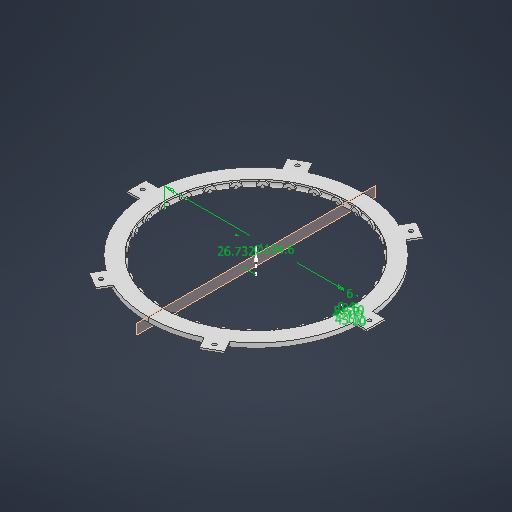
# Autodesk Inventor part: SAFRS-P-0034
Saved by Autodesk Inventor 2026.2 (Build 302298000, 298)
## iProperties
Created: 2025-12-01
Part Number: SAFRS-P-0034
Material: 일반
Document SubType Name: Modeling
Designer: jaewook
Density: 1 g/cm^3
Appearance: 기본값
Author: jaewook
Title: Fixer V1
Autodesk Inventor part; units mm, degrees
ref_plane "XZ Plane" through (0, 0, 0) normal (0, 1, 0) x (-1, 0, 0)
ref_plane "XY Plane" through (0, 0, 0) normal (0, 0, 1) x (1, 0, 0)
sketch "스케치1" plane through (0, 0, 0) normal (0, 0, 1) x (1, 0, 0)
  line L0 (0, 13.366) -> (0, -13.366)
  line L1 (98.7799, 5) -> (104.7799, 5)
  line L2 (104.7799, 5) -> (104.7799, -5)
  line L3 (104.7799, -5) -> (98.7799, -5)
  line L4 (98.7799, -5) -> (98.7799, 5)
  circle A0 centre (99.2799, 0) radius 3.1
  line L5 (99.2799, 0) -> (96.1799, 0)
  line L6 (96.1799, 7.3721) -> (96.1799, -2.237) construction
  line L7 (96.5799, 5) -> (96.5799, 1.5232)
  line L8 (96.5799, 5) -> (98.7799, 5)
  line L9 (99.7799, -5) -> (99.7799, -3.0594)
  circle A1 centre (99.2799, 0) radius 2.8 construction
  line L10 (99.3622, -4.0421) -> (90.1233, 5.1968) construction
  line L11 (99.2799, 0) -> (97.3, -1.9799) construction
  line L12 (104.7799, 0) -> (114.7799, 0)
  line L13 (114.7799, 0) -> (114.7799, 5)
  line L14 (114.7799, 5) -> (104.7799, 5)
  line L15 (104.7799, 5) -> (104.7799, 0)
  line L16 (99.7799, -3.0594) -> (101.7205, -5)
  point P0 (0, 0)
  point P1 (0, 0)
  point P2 (98.7799, 3.0594)
  dimension "d19" = 5.6
  dimension "d0" = 26.732
  dimension "d1" = 6.2
  dimension "d2" = 0.5
  dimension "d3" = 1
  dimension "d4" = 10
  dimension "d5" = 6
  dimension "d6" = 0.4
  dimension "d20" = 194.6
  dimension "d21" = 45
  dimension "d22" = 10
  dimension "d29" = 45
  constraints: 34 end point, 4 parallel, 4 vertical, 3 horizontal, 3 perpendicular, 3 point on circle, 3 point on line, 2 coincident, 2 horizontal alignment, 2 midpoint, 1 centre point, 1 collinear, 1 tangent, 4 other
  measures "d0" distance of L0.end L0.start
  measures "d1" diameter of A0
  measures "d2" distance from line of L5.start L4
  measures "d3" distance between parallel lines of L9 L4
  measures "d4" distance of L1.end L2.end
  measures "d5" distance of L1.start L1.end
  measures "d6" distance between parallel lines of L7 L6
  measures "d20" diameter of L11.end L0
  measures "d21" angle of L11 L5
  measures "d22" distance of L13.end L14.end
  measures "d29" angle of L3 L16
revolve "회전1" add sketch "스케치1" angle 360 about axis through (0, 13.366, 0) along (0, -1, 0) contours L1 L2 L3 L16 A0 L4 | L14 L13 L12 L2
revolve "회전2" add sketch "스케치1" angle 180 mid plane about axis through (99.2799, 0, 0) along (-1, 0, 0) contours L4 A0 L7 L8
pattern_circular "원형 패턴1" count 30 over 360 about axis through (0, -10, 0) along (0, 1, 0) of "회전2"
sketch "스케치7" plane through (0, 5, 0) normal (0, 1, 0) x (1, 0, 0)
  arc A0 (96.6213, -20.5375) -> (98.7799, 0) centre (0, 0) ccw projected
  circle A1 centre (0, 0) radius 114.7799 projected
  line L0 (114.7799, -10) -> (127.7799, -10)
  line L1 (127.7799, -10) -> (127.7799, 10)
  line L2 (127.7799, 10) -> (114.7799, 10)
  line L3 (114.7799, 10) -> (114.7799, -10) construction
  line L4 (114.7799, -10) -> (127.7799, 10) construction
  line L5 (127.7799, -10) -> (114.7799, 10) construction
  line L6 (114.7799, 10) -> (114.3435, 10)
  line L7 (114.7799, -10) -> (114.3435, -10)
  point P0 (121.2799, 0)
  dimension "d41" = 13
  dimension "d42" = 20
  constraints: 16 end point, 3 horizontal, 2 midpoint, 2 parallel, 2 point on circle, 1 horizontal alignment, 1 perpendicular, 1 tangent
  measures "d41" distance of L2.end L1.end
  measures "d42" distance of L1.end L0.end
extrude "돌출2" add sketch "스케치7" against normal blind 2 contours A1 L6 L2 L1 L0 L7
sketch "스케치3" plane through (0, 0, 0) normal (0, -1, 0) x (1, 0, 0)
  circle A0 centre (121.0617, 0) radius 2
  line L0 (127.7799, -10) -> (114.3435, -10) projected
  line L1 (127.7799, 10) -> (127.7799, -10) projected
  line L2 (114.3435, 10) -> (127.7799, 10) projected
  line L3 (114.3435, 10) -> (127.7799, -10) construction
  line L4 (114.3435, -10) -> (127.7799, 10) construction
  dimension "d23" = 4
  constraints: 4 end point, 2 coincident, 1 centre point, 1 midpoint
  measures "d23" diameter of A0
extrude "돌출1" cut sketch "스케치3" against normal through all
pattern_circular "원형 패턴3" count 6 over 360 about axis through (0, -10, 0) along (0, 1, 0) of "돌출1", "돌출2"
sketch "스케치2" plane through (0, 0, 0) normal (0, 0, 1) x (1, 0, 0)
  circle A0 centre (99.2799, 0) radius 3.1 projected
  circle A1 centre (99.2799, 0) radius 2.8
  line L0 (99.2799, -2.8) -> (99.2799, 2.8)
  line L1 (100.192, -3.6136) -> (93.7956, -0.336)
  line L2 (100.192, -3.6136) -> (94.0407, -3.6136)
  point P0 (0, 0)
  point P1 (98.003, -2.4919)
  dimension "d13" = 5.6
  dimension "d18" = 98.003
  constraints: 6 end point, 3 point on circle, 1 centre point, 1 coincident, 1 horizontal, 1 midpoint, 1 point on line, 1 tangent, 1 vertical
  measures "d13" diameter of A1
  measures "d18" horizontal distance of point (0, 0) point (98.003, -2.492)
revolve "회전3" add sketch "스케치2" angle 360 about axis through (99.2799, -2.8, 0) along (0, 1, 0) separate body picked at (100.5362, -0.405) contours A1 L0
pattern_circular "원형 패턴2" count 30 over 360 about axis through (0, -10, 0) along (0, 1, 0) of "회전3" bodies 2
sketch "스케치5" plane through (0, 0, 0) normal (1, 0, 0) x (0, 1, 0)
  line L0 (0, 114.7799) -> (0, -114.7799) projected
  line L1 (0, -104.7799) -> (-5, -104.7799) projected
  line L2 (0, -104.7799) -> (-5, -104.7799) projected
  line L3 (-5, -104.7799) -> (0, -111.8458)
  point P0 (0, 0)
  constraints: 2 end point, 1 point on line
revolve "회전4" add sketch "스케치5" angle 60 mid plane about axis through (0, 13.366, 0) along (0, -1, 0) bodies 1
pattern_circular "원형 패턴4" count 6 over 360 about axis through (0, -10, 0) along (0, 1, 0) of "회전4" bodies 1
split body "분할1" result two bodies by plane through (0, 0, 0) normal (1, 0, 0) bodies 1 first body at (95.212, 4.5, 53.6438)
